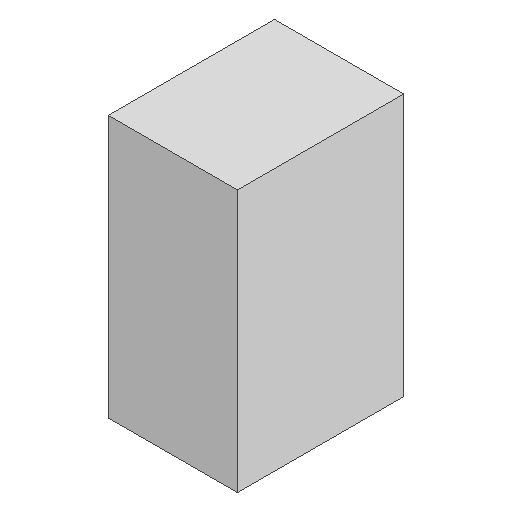
# Autodesk Inventor part: plug-demo
Saved by Autodesk Inventor 2026.1 (Build 301233020, 233B)
## iProperties
Created: 2025-11-10
Part Number: plug-demo
Material: Generic
Document SubType Name: Modeling
Designer: e3d
Density: 1 g/cm^3
Appearance: Default
Author: e3d
Autodesk Inventor part; units mm, degrees
ref_plane "YZ Plane" through (0, 0, 0) normal (1, 0, 0) x (0, 1, 0)
ref_plane "XZ Plane" through (0, 0, 0) normal (0, 1, 0) x (-1, 0, 0)
ref_plane "XY Plane" through (0, 0, 0) normal (0, 0, 1) x (1, 0, 0)
sketch "Sketch1" plane through (0, 0, 0) normal (0, 1, 0) x (-1, 0, 0)
  line L0 (6.5131, 7.6247) -> (-6.0061, 7.6247)
  line L1 (-6.0061, 7.6247) -> (-6.0061, -8.4827)
  line L2 (-6.0061, -8.4827) -> (6.5131, -8.4827)
  line L3 (6.5131, -8.4827) -> (6.5131, 7.6247)
  point P0 (0, 0)
  constraints: 8 end point, 2 parallel, 1 horizontal, 1 perpendicular
extrude "Extrusion1" add sketch "Sketch1" along normal blind 25.4
equation "\"Width\" = 50.8"
equation "\"Length\" = 76.2"
equation "\"Height\" = 101.6"
body "Solid1"
